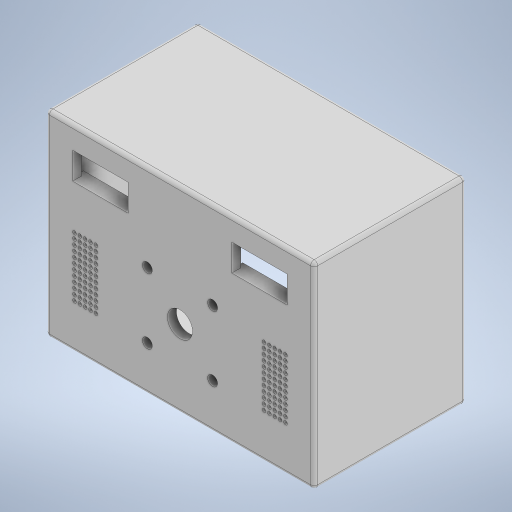
# Autodesk Inventor part: case_1
Saved by Autodesk Inventor 2024 (Build 280153000, 153)
## iProperties
Created: 2026-02-20
Part Number: case_1
Material: Generic
Document SubType Name: Modeling
Designer: janst
Density: 1 g/cm^3
Appearance: Default
Author: janst
## iProperties of the stored document case_1_3DPrint.ipt
Created: 2026-02-20
Part Number: case_1_3DPrint
Material: Generic
Document SubType Name: Modeling
Designer: janst
Density: 1 g/cm^3
Appearance: Default
Author: janst
Autodesk Inventor part; units mm, degrees
ref_plane "YZ Plane" through (0, 0, 0) normal (1, 0, 0) x (0, 1, 0)
ref_plane "XZ Plane" through (0, 0, 0) normal (0, 1, 0) x (-1, 0, 0)
ref_plane "XY Plane" through (0, 0, 0) normal (0, 0, 1) x (1, 0, 0)
sketch "Sketch1" plane through (0, 0, 0) normal (0, 0, 1) x (1, 0, 0)
  line L0 (75, -55) -> (-75, -55)
  line L1 (-75, -55) -> (-75, 55)
  line L2 (-75, 55) -> (75, 55)
  line L3 (75, 55) -> (75, -55)
  line L4 (75, -55) -> (-75, 55) construction
  line L5 (-75, -55) -> (75, 55) construction
  line L6 (18.25, -30) -> (-18.25, -30)
  line L7 (-18.25, -30) -> (-18.25, 6.5)
  line L8 (-18.25, 6.5) -> (18.25, 6.5)
  line L9 (18.25, 6.5) -> (18.25, -30)
  line L10 (18.25, -30) -> (-18.25, 6.5) construction
  line L11 (-18.25, -30) -> (18.25, 6.5) construction
  line L12 (0, -77) -> (0, 77) projected
  line L13 (-29, 27.5) -> (-60, 27.5)
  line L14 (-60, 27.5) -> (-60, 42.5)
  line L15 (-60, 42.5) -> (-29, 42.5)
  line L16 (-29, 42.5) -> (-29, 27.5)
  line L17 (-29, 27.5) -> (-60, 42.5) construction
  line L18 (-60, 27.5) -> (-29, 42.5) construction
  circle A0 centre (0, -11.75) radius 7
  line L19 (60, 27.5) -> (29, 27.5)
  line L20 (29, 27.5) -> (29, 42.5)
  line L21 (29, 42.5) -> (60, 42.5)
  line L22 (60, 42.5) -> (60, 27.5)
  line L23 (60, 27.5) -> (29, 42.5) construction
  line L24 (29, 27.5) -> (60, 42.5) construction
  line L25 (-75, 35) -> (75, 35)
  point P0 (0, 0)
  point P1 (0, -11.75)
  point P2 (-44.5, 35)
  point P3 (44.5, 35)
  dimension "d0" = 110
  dimension "d1" = 150
  dimension "d2" = 36.5
  dimension "d3" = 36.5
  dimension "d4" = 25
  dimension "d5" = 14
  dimension "d6" = 31
  dimension "d7" = 15
  dimension "d8" = 15
  dimension "d9" = 31
  dimension "d11" = 20
  dimension "d12" = 15
  dimension "d13" = 15
  constraints: 50 end point, 9 parallel, 8 midpoint, 5 coincident, 5 point on line, 4 horizontal, 4 perpendicular, 1 centre point
  measures "d0" distance of L2.end L0.start
  measures "d1" distance of L1.end L2.end
  measures "d2" distance of L8.end L6.start
  measures "d3" distance of L6.start L6.end
  measures "d4" distance between parallel lines of L0 L6
  measures "d5" diameter of A0
  measures "d6" distance of L13.start L13.end
  measures "d7" distance of L15.end L13.start
  measures "d8" distance of L19.end L20.end
  measures "d9" distance of L19.start L19.end
  measures "d11" distance between parallel lines of L2 L25
  measures "d12" distance between parallel lines of L1 L14
  measures "d13" distance between parallel lines of L3 L22
extrude "Extrusion1" add sketch "Sketch1" against normal blind 5
extrude "Extrusion2" cut sketch "Sketch1" against normal blind 5 contours L25 L20 L21 L22 | L22 L19 L20 L25 | A0 L12 | L12 A0 | L25 L16 L13 L14 | L14 L15 L16 L25
hole "Hole1" at (-18.25, 6.5, 0) at (-18.25, -30, 0) at (18.25, -30, 0) at (18.25, 6.5, 0) direction (0, 0, -1) diameter 5.5 end through all
sketch "Sketch2" plane through (0, 0, -5) normal (0, 0, -1) x (-1, 0, 0)
  circle A0 centre (-18.25, 6.5) radius 2.75 projected
  circle A1 centre (-18.25, -30) radius 2.75 projected
  circle A2 centre (18.25, -30) radius 2.75 projected
  circle A3 centre (18.25, 6.5) radius 2.75 projected
  circle A4 centre (0, -11.75) radius 7 projected
  line L0 (-29, 27.5) -> (-60, 27.5) projected
  line L1 (-60, 27.5) -> (-60, 42.5) projected
  line L2 (-60, 42.5) -> (-29, 42.5) projected
  line L3 (-29, 42.5) -> (-29, 27.5) projected
  line L4 (29, 42.5) -> (60, 42.5) projected
  line L5 (60, 42.5) -> (60, 27.5) projected
  line L6 (60, 27.5) -> (29, 27.5) projected
  line L7 (29, 27.5) -> (29, 42.5) projected
  line L8 (75, 55) -> (-75, 55) projected
  line L9 (-75, 55) -> (-75, -55) projected
  line L10 (-75, -55) -> (75, -55) projected
  line L11 (75, -55) -> (75, 55) projected
  line L12 (-27, 44.5) -> (-62, 44.5)
  line L13 (-62, 44.5) -> (-62, 25.5)
  line L14 (-62, 25.5) -> (-27, 25.5)
  line L15 (-27, 25.5) -> (-27, 44.5)
  line L16 (62, 44.5) -> (27, 44.5)
  line L17 (27, 44.5) -> (27, 25.5)
  line L18 (27, 25.5) -> (62, 25.5)
  line L19 (62, 25.5) -> (62, 44.5)
  line L20 (-62, 42.5) -> (-27, 42.5)
  line L21 (-62, 27.5) -> (-27, 27.5)
  line L22 (27, 42.5) -> (62, 42.5)
  line L23 (62, 27.5) -> (27, 27.5)
  line L24 (-60, 42.5) -> (-29, 42.5) projected
  line L25 (-29, 27.5) -> (-60, 27.5) projected
  line L26 (29, 42.5) -> (60, 42.5) projected
  point P0 (0, 0)
  dimension "d25" = 2
  dimension "d26" = 2
  constraints: 24 end point, 9 point on line, 3 collinear, 3 parallel, 1 perpendicular, 6 other
  measures "d25" distance between parallel lines of L15 L3
  measures "d26" distance between parallel lines of L17 L7
extrude "Extrusion3" add sketch "Sketch2" along normal blind 3 contours L21 L15 L14 L13 L0 | L2 L20 L13 L12 L15 | L22 L17 L16 L19 L4 | L6 L23 L19 L18 L17
sketch "Sketch5" plane through (0, 0, -5) normal (0, 0, -1) x (-1, 0, 0)
  line L0 (-62, 27.5) -> (-60, 27.5) projected
  line L1 (-60, 27.5) -> (-60, 42.5) projected
  line L2 (-60, 42.5) -> (-62, 42.5) projected
  line L3 (-62, 42.5) -> (-62, 44.5) projected
  line L4 (-62, 44.5) -> (-27, 44.5) projected
  line L5 (-27, 44.5) -> (-27, 42.5) projected
  line L6 (-27, 42.5) -> (-29, 42.5) projected
  line L7 (-29, 42.5) -> (-29, 27.5) projected
  line L8 (-29, 27.5) -> (-27, 27.5) projected
  line L9 (-27, 27.5) -> (-27, 25.5) projected
  line L10 (-27, 25.5) -> (-62, 25.5) projected
  line L11 (-62, 25.5) -> (-62, 27.5) projected
  line L12 (27, 27.5) -> (29, 27.5) projected
  line L13 (29, 27.5) -> (29, 42.5) projected
  line L14 (29, 42.5) -> (27, 42.5) projected
  line L15 (27, 42.5) -> (27, 44.5) projected
  line L16 (27, 44.5) -> (62, 44.5) projected
  line L17 (62, 44.5) -> (62, 42.5) projected
  line L18 (62, 42.5) -> (60, 42.5) projected
  line L19 (60, 42.5) -> (60, 27.5) projected
  line L20 (60, 27.5) -> (62, 27.5) projected
  line L21 (62, 27.5) -> (62, 25.5) projected
  line L22 (62, 25.5) -> (27, 25.5) projected
  line L23 (27, 25.5) -> (27, 27.5) projected
  circle A0 centre (-18.25, 6.5) radius 2.75 projected
  circle A1 centre (-18.25, -30) radius 2.75 projected
  circle A2 centre (18.25, -30) radius 2.75 projected
  circle A3 centre (18.25, 6.5) radius 2.75 projected
  circle A4 centre (0, -11.75) radius 7 projected
  line L24 (75, 55) -> (-75, 55) projected
  line L25 (-75, 55) -> (-75, -55) projected
  line L26 (-75, -55) -> (75, -55) projected
  line L27 (75, -55) -> (75, 55) projected
  line L28 (-63, 45.5) -> (-24, 45.5)
  line L29 (-24, 45.5) -> (-24, 23.5)
  line L30 (-24, 23.5) -> (-63, 23.5)
  line L31 (-63, 23.5) -> (-63, 45.5)
  line L32 (-27, 27.5) -> (-62, 27.5) projected
  line L33 (62, 27.5) -> (27, 27.5) projected
  line L34 (27, 42.5) -> (62, 42.5) projected
  line L35 (26, 23.5) -> (65, 23.5)
  line L36 (65, 23.5) -> (65, 45.5)
  line L37 (65, 45.5) -> (26, 45.5)
  line L38 (26, 45.5) -> (26, 23.5)
  line L39 (-62, 42.5) -> (-27, 42.5) projected
  point P0 (0, 0)
  dimension "d34" = 3
  dimension "d35" = 5
  dimension "d36" = 4
  dimension "d42" = 3
  dimension "d43" = 5
  dimension "d44" = 4
  dimension "d45" = 3
  dimension "d46" = 3
  constraints: 16 end point, 8 coincident, 4 parallel, 2 horizontal, 2 perpendicular
  measures "d34" distance between parallel lines of L31 L1
  measures "d35" distance between parallel lines of L29 L7
  measures "d36" distance between parallel lines of L30 L32
  measures "d42" distance between parallel lines of L38 L13
  measures "d43" distance between parallel lines of L36 L19
  measures "d44" distance between parallel lines of L35 L33
  measures "d45" distance between parallel lines of L37 L34
  measures "d46" distance between parallel lines of L28 L39
hole "Hole2" at (24, 45.5, -5) at (63, 45.5, -5) at (63, 23.5, -5) at (24, 23.5, -5) at (-26, 23.5, -5) at (-26, 45.5, -5) at (-65, 45.5, -5) at (-65, 23.5, -5) direction (0, 0, 1) diameter 2.2 depth 3 tip angle 118
sketch "Sketch6" plane through (0, 0, -5) normal (0, 0, -1) x (-1, 0, 0)
  circle A0 centre (65, 23.5) radius 1.1 projected
  circle A1 centre (65, 45.5) radius 1.1 projected
  circle A2 centre (26, 45.5) radius 1.1 projected
  circle A3 centre (26, 23.5) radius 1.1 projected
  circle A4 centre (-24, 23.5) radius 1.1 projected
  circle A5 centre (-63, 23.5) radius 1.1 projected
  circle A6 centre (-63, 45.5) radius 1.1 projected
  circle A7 centre (-24, 45.5) radius 1.1 projected
  line L0 (-62, 27.5) -> (-60, 27.5) projected
  line L1 (-60, 27.5) -> (-60, 42.5) projected
  line L2 (-60, 42.5) -> (-62, 42.5) projected
  line L3 (-62, 42.5) -> (-62, 44.5) projected
  line L4 (-62, 44.5) -> (-27, 44.5) projected
  line L5 (-27, 44.5) -> (-27, 42.5) projected
  line L6 (-27, 42.5) -> (-29, 42.5) projected
  line L7 (-29, 42.5) -> (-29, 27.5) projected
  line L8 (-29, 27.5) -> (-27, 27.5) projected
  line L9 (-27, 27.5) -> (-27, 25.5) projected
  line L10 (-27, 25.5) -> (-62, 25.5) projected
  line L11 (-62, 25.5) -> (-62, 27.5) projected
  line L12 (27, 27.5) -> (29, 27.5) projected
  line L13 (29, 27.5) -> (29, 42.5) projected
  line L14 (29, 42.5) -> (27, 42.5) projected
  line L15 (27, 42.5) -> (27, 44.5) projected
  line L16 (27, 44.5) -> (62, 44.5) projected
  line L17 (62, 44.5) -> (62, 42.5) projected
  line L18 (62, 42.5) -> (60, 42.5) projected
  line L19 (60, 42.5) -> (60, 27.5) projected
  line L20 (60, 27.5) -> (62, 27.5) projected
  line L21 (62, 27.5) -> (62, 25.5) projected
  line L22 (62, 25.5) -> (27, 25.5) projected
  line L23 (27, 25.5) -> (27, 27.5) projected
  circle A8 centre (-18.25, 6.5) radius 2.75 projected
  circle A9 centre (-18.25, -30) radius 2.75 projected
  circle A10 centre (18.25, -30) radius 2.75 projected
  circle A11 centre (18.25, 6.5) radius 2.75 projected
  circle A12 centre (0, -11.75) radius 7 projected
  line L24 (75, 55) -> (-75, 55) projected
  line L25 (-75, 55) -> (-75, -55) projected
  line L26 (-75, -55) -> (75, -55) projected
  line L27 (75, -55) -> (75, 55) projected
  line L28 (-65, 18.5) -> (-40.5, 18.5)
  line L29 (-40.5, 18.5) -> (-40.5, -45)
  line L30 (-40.5, -45) -> (-65, -45)
  line L31 (-65, -45) -> (-65, 18.5)
  line L32 (40.5, 18.5) -> (65, 18.5)
  line L33 (65, 18.5) -> (65, -45)
  line L34 (65, -45) -> (40.5, -45)
  line L35 (40.5, -45) -> (40.5, 18.5)
  circle A13 centre (-59, -30) radius 1
  point P0 (0, 0)
  dimension "d54" = 24.5
  dimension "d55" = 24.5
  dimension "d56" = 63.5
  dimension "d57" = 63.5
  dimension "d58" = 10
  dimension "d59" = 10
  dimension "d60" = 10
  dimension "d61" = 10
  dimension "d65" = 2
  dimension "d66" = 15
  dimension "d67" = 6
  constraints: 16 end point, 8 coincident, 4 parallel, 2 horizontal, 2 perpendicular, 1 centre point
  measures "d54" distance of L28.start L28.end
  measures "d55" distance of L32.start L32.end
  measures "d56" distance of L28.end L29.end
  measures "d57" distance of L32.end L33.end
  measures "d58" distance between parallel lines of L26 L30
  measures "d59" distance between parallel lines of L25 L31
  measures "d60" distance between parallel lines of L27 L33
  measures "d61" distance between parallel lines of L26 L34
  measures "d65" diameter of A13
  measures "d66" distance from line of L30 A13.centre
  measures "d67" distance from line of L31 A13.centre
extrude "Extrusion5" cut sketch "Sketch6" against normal blind 10 contours A13
pattern_linear "Rectangular Pattern1" count 5 spacing 3 along (-1, 0, 0) count 12 spacing 3 along (0, 1, 0) of "Extrusion5"
pattern_linear "Rectangular Pattern2" count 2 spacing 106 along (-1, 0, 0) of "Extrusion5", "Rectangular Pattern1"
hole "Hole3" at (65, -45, -5) at (40.5, -45, -5) at (40.5, 18.5, -5) at (65, 18.5, -5) at (-40.5, 18.5, -5) at (-65, 18.5, -5) at (-65, -45, -5) at (-40.5, -45, -5) direction (0, 0, 1) diameter 2.2 depth 3 tip angle 118
sketch "Sketch3" plane through (0, 0, -5) normal (0, 0, -1) x (-1, 0, 0)
  line L0 (75, 55) -> (-75, 55) projected
  line L1 (-75, 55) -> (-75, -55) projected
  line L2 (-75, -55) -> (75, -55) projected
  line L3 (75, -55) -> (75, 55) projected
  line L4 (-70, 50) -> (70, 50)
  line L5 (70, 50) -> (70, -50)
  line L6 (70, -50) -> (-70, -50)
  line L7 (-70, -50) -> (-70, 50)
  point P0 (0, 0)
  dimension "d29" = 5
  constraints: 8 end point, 3 other
  measures "d29" distance between parallel lines of L0 L4
extrude "Extrusion4" add sketch "Sketch3" along normal blind 80
fillet "Fillet1" radius 2 16 edges at (75, 55, -42.5) (75, -55, -42.5) (75, 0, 0) (75, 0, -85) (0, -55, 0) (-75, 0, 0) (0, 55, 0) (-75, 55, -42.5) (-75, -55, -42.5) (-75, 0, -85) (0, 55, -85) (0, -55, -85) (-70, 0, -85) (0, 50, -85) (0, -50, -85) (70, 0, -85)
equation "\"d3\" = d2"
equation "\"d8\" = d7"
equation "\"d9\" = d6"
equation "\"d13\" = d12"
equation "\"d26\" = d25"
equation "\"d42\" = d34"
equation "\"d43\" = d35"
equation "\"d44\" = d36"
equation "\"d45\" = d37"
equation "\"d55\" = d54"
equation "\"d57\" = d56"
equation "\"d60\" = d59"
equation "\"d61\" = d58"
equation "\"d37\" = 3"
body "Solid1"
